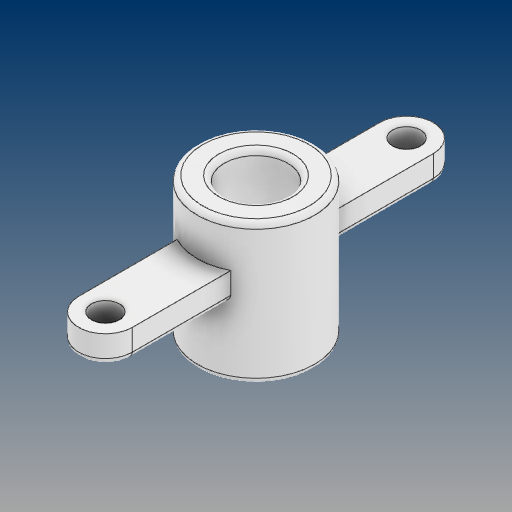
# Autodesk Inventor part: 05_Tam_truot_lo_xo
Saved by Autodesk Inventor 2021 (Build 250183000, 183)
## iProperties
Created: 2024-04-07
Part Number: 05_Tam_truot_lo_xo
Material: ABS Plastic
Document SubType Name: Modeling
Designer: Admin
Density: 1.06 g/cm^3
Appearance: Smooth - White
Author: Admin
Autodesk Inventor part; units mm, degrees
ref_plane "YZ Plane" through (0, 0, 0) normal (1, 0, 0) x (0, 1, 0)
ref_plane "XZ Plane" through (0, 0, 0) normal (0, 1, 0) x (-1, 0, 0)
ref_plane "XY Plane" through (0, 0, 0) normal (0, 0, 1) x (1, 0, 0)
sketch "Sketch1" plane through (0, 0, 0) normal (0, 1, 0) x (-1, 0, 0)
  line L0 (0, 28) -> (0, -28) construction
  line L1 (-5, 28) -> (-5, -28)
  line L2 (5, -28) -> (5, 28)
  arc A0 (5, 28) -> (-5, 28) centre (0, 28) ccw
  arc A1 (-5, -28) -> (5, -28) centre (0, -28) ccw
  circle A2 centre (0, 0) radius 5.9
  circle A3 centre (0, 0) radius 10.9
  circle A4 centre (0, 0) radius 3.5
  point P0 (-5, 9.6856)
  point P1 (-5, -9.6856)
  point P2 (5, -9.6856)
  point P3 (5, 9.6856)
  dimension "d0" = 56
  dimension "d1" = 5
  dimension "d2" = 11.8
  dimension "d3" = 5
  dimension "d10" = 7
  constraints: 8 end point, 5 centre point, 4 point on circle, 4 tangent, 3 coincident, 1 midpoint, 1 parallel, 1 vertical
  measures "d0" distance of L0.start L0.end
  measures "d1" radius of A1
  measures "d2" diameter of A2
  measures "d3" radial gap between concentric circles of A2 A3
  measures "d10" diameter of A4
extrude "Extrusion1" add sketch "Sketch1" against normal blind 5
extrude "Extrusion2" cut sketch "Sketch1" against normal blind 18.25 contours A4
extrude "Extrusion3" add sketch "Sketch1" along normal blind 8 contours A3 L2 A2 L1 | L1 A2 A3 | A3 L2 A2 | L1 A2 L2 A3
sketch "Sketch2" plane through (0, -5, 0) normal (0, -1, 0) x (1, 0, 0)
  line L0 (5, -28) -> (5, -9.6856) projected
  arc A0 (5, -9.6856) -> (5, 9.6856) centre (0, 0) ccw projected
  line L1 (5, 9.6856) -> (5, 28) projected
  arc A1 (5, 28) -> (-5, 28) centre (0, 28) ccw projected
  line L2 (-5, 28) -> (-5, 9.6856) projected
  arc A2 (-5, 9.6856) -> (-5, -9.6856) centre (0, 0) ccw projected
  line L3 (-5, -9.6856) -> (-5, -28) projected
  arc A3 (-5, -28) -> (5, -28) centre (0, -28) ccw projected
  circle A4 centre (0, 0) radius 3.5 projected
hole "Hole1" at (0, -5, 28) at (0, -5, -28) direction (0, 1, 0) diameter 5.2 end through all
sketch "Sketch3" plane through (0, -5, 0) normal (0, -1, 0) x (1, 0, 0)
  arc A0 (5, -9.6856) -> (5, 9.6856) centre (0, 0) ccw projected
  circle A1 centre (0, 0) radius 5.9 projected
extrude "Extrusion4" cut sketch "Sketch3" against normal blind 28
sketch "Sketch4" plane through (0, -5, 0) normal (0, -1, 0) x (1, 0, 0)
  arc A0 (-5, 9.6856) -> (-5, -9.6856) centre (0, 0) ccw projected
  line L0 (-5, 28) -> (-5, 9.6856) projected
  circle A1 centre (0, 0) radius 10.9
  circle A2 centre (0, 0) radius 5.9 projected
  point P0 (-5, -9.6856)
  constraints: 1 coincident, 3 other
extrude "Extrusion5" add sketch "Sketch4" along normal blind 10
sketch "Sketch5" plane through (0, -15, 0) normal (0, -1, 0) x (1, 0, 0)
  circle A0 centre (0, 0) radius 10.9 projected
  circle A1 centre (0, 0) radius 3.25
  dimension "d23" = 6.5
  constraints: 1 centre point, 1 coincident
  measures "d23" diameter of A1
extrude "Extrusion6" add sketch "Sketch5" along normal blind 3
fillet "Fillet1" radius 1 8 edges at (10.9, 8, 0) (-10.9, -18, 0) (0, -5, -33) (5, -5, -18.8428) (-5, -5, -18.8428) (0, -5, 33) (5, -5, 18.8428) (-5, -5, 18.8428)
fillet "Fillet2" radius 1 2 edges at (0, 8, 5.9) (0, 8, -5.9)
chamfer "Chamfer1" distance 0.5 angle 45 2 edges at (-3.25, -15, 0) (-3.25, -18, 0)
body "Solid1"
